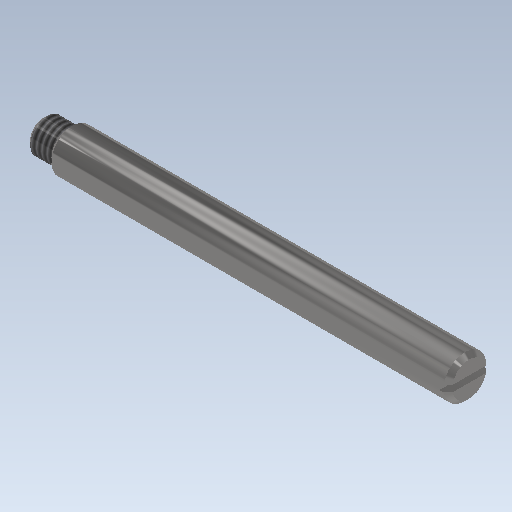
# Autodesk Inventor part: Shaft
Saved by Autodesk Inventor 2020.1 (Build 241239000, 239)
## iProperties
Created: 2015-12-25
Part Number: Shaft
Material: Steel
Document SubType Name: Modeling
Designer: User
Density: 7.85 g/cm^3
Appearance: Steel - Polished
Author: User
Autodesk Inventor part; units mm, degrees
ref_plane "YZ Plane" through (0, 0, 0) normal (1, 0, 0) x (0, 1, 0)
ref_plane "XZ Plane" through (0, 0, 0) normal (0, 1, 0) x (-1, 0, 0)
ref_plane "XY Plane" through (0, 0, 0) normal (0, 0, 1) x (1, 0, 0)
sketch "Sketch1" plane through (0, 0, 0) normal (0, 0, 1) x (1, 0, 0)
  line L0 (0, 0) -> (0, 4)
  line L1 (0, 4) -> (6, 4)
  line L2 (7, 3.5) -> (7, 5)
  line L3 (7, 5) -> (100, 5)
  line L4 (100, 5) -> (100, 0)
  line L5 (100, 0) -> (0, 0)
  line L6 (6, 4) -> (6, 3.5)
  line L7 (6, 3.5) -> (7, 3.5)
  dimension "d0" = 8
  dimension "d1" = 10
  dimension "d3" = 100
  dimension "d17" = 7
  dimension "d18" = 1
  dimension "d19" = 7
  constraints: 16 end point, 3 parallel, 3 vertical, 1 horizontal, 1 perpendicular
  measures "d0" diameter of L1 L5
  measures "d1" diameter of L3 L5
  measures "d3" distance between parallel lines of L4 L0
  measures "d17" distance between parallel lines of L0 L2
  measures "d18" distance between parallel lines of L2 L6
  measures "d19" diameter of L7 L5
revolve "Revolution1" add sketch "Sketch1" angle 360 about axis through (100, 0, 0) along (-1, 0, 0)
thread "Thread1" size "M8x1.25" class "6g" standard "ISO Metric profile" full length
chamfer "Chamfer1" distance 1 angle 45 1 edges at (0, -4, 0)
sketch "Sketch2" plane through (0, 0, 0) normal (0, 0, 1) x (1, 0, 0)
  line L0 (100, 0.75) -> (98, 0.75)
  line L1 (98, 0.75) -> (98, -0.75)
  line L2 (98, -0.75) -> (100, -0.75)
  line L3 (100, -0.75) -> (100, 0.75)
  line L4 (100, -5) -> (100, 5) construction
  point P0 (0, 0)
  point P1 (98, 0)
  dimension "d10" = 1.5
  dimension "d11" = 2
  constraints: 8 end point, 2 parallel, 1 collinear, 1 horizontal, 1 horizontal alignment, 1 midpoint, 1 perpendicular
  measures "d10" distance between parallel lines of L2 L0
  measures "d11" distance of L0.start L0.end
extrude "Extrusion1" cut sketch "Sketch2" along normal through all both and the other way through all
chamfer "Chamfer2" distance 1 angle 45 3 edges at (100, -5, 0) (100, 3.7914, -3.2596) (100, 3.7914, 3.2596)
body "Solid1"
